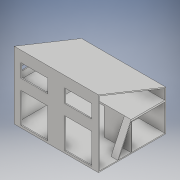
# Autodesk Inventor part: out
Saved by Autodesk Inventor 2017 (Build 210142000, 142)
## iProperties
Created: 2019-10-04
Part Number: out
Material: Generic
Document SubType Name: Modeling
Designer: Ellie
Density: 1 g/cm^3
Appearance: Default
Author: Ellie
Autodesk Inventor part; units mm, degrees
ref_plane "YZ Plane" through (0, 0, 0) normal (1, 0, 0) x (0, 1, 0)
ref_plane "XZ Plane" through (0, 0, 0) normal (0, 1, 0) x (-1, 0, 0)
sketch "Sketch1" plane through (0, 0, 0) normal (0, 1, 0) x (-1, 0, 0)
  line L0 (-3048, 3810) -> (3048, 3810)
  line L1 (3048, 3810) -> (3048, -3810)
  line L2 (3048, -3810) -> (-3048, -3810)
  line L3 (-3048, -3810) -> (-3048, 3810)
  line L4 (-3048, 3810) -> (3048, -3810) construction
  line L5 (3048, 3810) -> (-3048, -3810) construction
  point P0 (0, 0)
  dimension "d0" = 7620
  dimension "d1" = 6096
  constraints: 12 end point, 2 midpoint, 2 parallel, 1 horizontal, 1 perpendicular
  measures "d0" distance of L0.end L1.end
  measures "d1" distance of L1.end L2.end
extrude "main body" add sketch "Sketch1" along normal blind 3657.6
sketch "Sketch3" plane through (0, 0, 0) normal (0, 0, 1) x (1, 0, 0)
  line L0 (-3048, 3657.6) -> (-3048, 6096)
  line L1 (-3048, 6096) -> (3048, 3657.6)
  line L2 (3048, 3657.6) -> (-3048, 3657.6)
  point P0 (0, 0)
  dimension "d4" = 2438.4
  constraints: 6 end point, 2 coincident, 1 vertical
  measures "d4" distance of L0.start L0.end
extrude "triangle" add sketch "Sketch3" along normal mid plane 7620
shell "Shell1" thickness 88.9 removed faces 1 at (-1016, 3251.2, 3810)
ref_plane "Work Plane1" through (-2959.1, 2527.3, 3810) normal (0, 1, 0) x (1, 0, 0)
sketch "Sketch6" plane through (-2959.1, 2527.3, 3810) normal (0, 1, 0) x (1, 0, 0)
  line L0 (5918.2, 0) -> (2870.2, 0)
  line L1 (2870.2, 0) -> (2870.2, 7531.1)
  line L2 (2870.2, 7531.1) -> (5918.2, 7531.1)
  line L3 (5918.2, 7531.1) -> (5918.2, 0)
  point P0 (2959.1, 3810)
  dimension "d12" = 3048
  constraints: 8 end point, 2 parallel, 1 coincident, 1 horizontal, 1 perpendicular
  measures "d12" distance of L0.start L0.end
extrude "second floor" add sketch "Sketch6" along normal blind 152.4
ref_plane "Work Plane3" through (-2959.1, 3136.9, 3810) normal (0, 1, 0) x (1, 0, 0)
sketch "Sketch8" plane through (-2959.1, 3136.9, 3810) normal (0, 1, 0) x (1, 0, 0)
  line L0 (0, 7531.1) -> (2870.2, 7531.1)
  line L1 (2870.2, 7531.1) -> (2870.2, 5397.5)
  line L2 (2870.2, 5397.5) -> (0, 5397.5)
  line L3 (0, 5397.5) -> (0, 7531.1)
  line L4 (2870.2, 7531.1) -> (2870.2, 0) projected
  line L5 (0, 0) -> (0, 7531.1) projected
  line L6 (2870.2, 7531.1) -> (3479.8, 7531.1)
  line L7 (3479.8, 7531.1) -> (3479.8, 6616.7)
  line L8 (3479.8, 6616.7) -> (2870.2, 6616.7)
  line L9 (2870.2, 6616.7) -> (2870.2, 7531.1)
  point P0 (2959.1, 3810)
  dimension "d17" = 0
  dimension "d19" = 0
  dimension "d20" = 2133.6
  dimension "d23" = 0
  dimension "d39" = 609.6
  dimension "d40" = 914.4
  constraints: 16 end point, 4 parallel, 2 horizontal, 2 perpendicular, 1 collinear
  measures "d17" distance between parallel lines of L4 L1
  measures "d19" distance from line of L0 L5.end
  measures "d20" distance of L0.end L1.end
  measures "d23" distance between parallel lines of L5 L3
  measures "d39" distance of L7.end L8.end
  measures "d40" distance of L6.end L7.end
extrude "bedroom" add sketch "Sketch8" along normal blind 152.4
sketch "Sketch16" plane through (-88.9, 3136.9, -1587.5) normal (1, 0, 0) x (0, 0, -1)
  line L0 (1219.2, 0) -> (304.8, -457.2)
  line L1 (1219.2, 0) -> (1219.2, 152.4) projected
  line L2 (2133.6, -457.2) -> (-5397.5, -457.2) projected
  line L3 (0, 0) -> (0, 152.4) projected
  line L4 (1219.2, 152.4) -> (0, -457.2)
  line L5 (2133.6, -457.2) -> (-5397.5, -457.2) projected
  line L6 (304.8, -457.2) -> (0, -457.2)
  line L7 (1219.2, 152.4) -> (1219.2, 0)
  point P0 (-1587.5, -3136.9)
  point P1 (-1803.4, -558.8)
  point P2 (-5397.5, -457.2)
  dimension "d42" = 0
  constraints: 8 end point, 1 horizontal, 1 parallel, 1 vertical, 4 other
  measures "d42" distance from line of L3 L4.end
extrude "upper stairs" add sketch "Sketch16" along normal blind 609.6
sketch "Sketch17" plane through (-3048, 0, 3810) normal (0, 0, 1) x (1, 0, 0)
  line L0 (2959.1, 2527.3) -> (1822.0554, 88.9)
  line L1 (6007.1, 88.9) -> (88.9, 88.9) projected
  line L2 (2959.1, 2679.7) -> (1750.9901, 88.9)
  line L3 (6007.1, 2527.3) -> (2959.1, 2527.3) projected
  line L4 (3022.6, 2527.3) -> (3022.6, 25.4) projected
  line L5 (2959.1, 2679.7) -> (2959.1, 2527.3)
  line L6 (1750.9901, 88.9) -> (1822.0554, 88.9)
  line L7 (2959.1, 2679.7) -> (6007.1, 2679.7) projected
  line L8 (2959.1, 2527.3) -> (2959.1, 2679.7) projected
  line L9 (2959.1, 2679.7) -> (2959.1, 2527.3)
  point P0 (3048, 0)
  point P1 (88.9, 88.9)
  point P2 (3022.6, 25.4)
  dimension "d46" = 115
  constraints: 10 end point, 1 coincident, 1 collinear, 1 horizontal, 1 parallel, 1 vertical, 3 other
  measures "d46" angle of L3 L0
extrude "main stairs" add sketch "Sketch17" against normal blind 609.6 contours L0 L1 L2 L5
sketch "Sketch18" plane through (2959.1, 88.9, -3721.1) normal (-1, 0, 0) x (0, 0, 1)
  point P0 (3721.1, -88.9)
ref_plane "Work Plane4" through (0, 0, 1371.6) normal (0, 0, 1) x (1, 0, 0)
sketch "Sketch20" plane through (0, 0, 1371.6) normal (0, 0, 1) x (1, 0, 0)
  line L0 (2959.1, 2527.3) -> (-88.9, 2527.3) projected
  line L1 (2959.1, 88.9) -> (2959.1, 2527.3) projected
  line L2 (-88.9, 2527.3) -> (2959.1, 2527.3)
  line L3 (2959.1, 2527.3) -> (2959.1, 88.9)
  line L4 (2959.1, 88.9) -> (-88.9, 88.9)
  line L5 (-88.9, 88.9) -> (-88.9, 2527.3)
  point P0 (0, 0)
  constraints: 8 end point, 2 parallel, 1 horizontal, 1 perpendicular
extrude "room wall 1" add sketch "Sketch20" along normal blind 50.8
sketch "Sketch21" plane through (-88.9, 2679.7, -3721.1) normal (-1, 0, 0) x (0, 0, 1)
  line L0 (7531.1, -152.4) -> (5143.5, -152.4) projected
  line L1 (5143.5, -2590.8) -> (7531.1, -2590.8) projected
  line L2 (5143.5, -152.4) -> (7531.1, -152.4)
  line L3 (7531.1, -152.4) -> (7531.1, -2590.8)
  line L4 (7531.1, -2590.8) -> (5143.5, -2590.8)
  line L5 (5143.5, -2590.8) -> (5143.5, -152.4)
  line L6 (6921.5, -2590.8) -> (6921.5, 0) projected
  line L7 (5143.5, -152.4) -> (5143.5, -2590.8) projected
  point P0 (3721.1, -2679.7)
  constraints: 8 end point, 3 parallel, 2 point on line, 1 horizontal
extrude "room wall 2" add sketch "Sketch21" against normal blind 50.8
sketch "Sketch23" plane through (-3048, 0, 3810) normal (0, 0, 1) x (1, 0, 0)
  line L0 (0, 0) -> (0, 6096) projected
  line L1 (6096, 0) -> (6096, 3657.6) projected
  line L2 (0, 6096) -> (6096, 3657.6)
  line L3 (6096, 3657.6) -> (6096, 0)
  line L4 (6096, 0) -> (0, 0) projected
  line L5 (6096, 0) -> (0, 0)
  line L6 (6096, 3657.6) -> (0, 6096) projected
  line L7 (0, 0) -> (0, 6096)
  line L8 (1750.9901, 88.9) -> (88.9, 88.9) projected
  point P0 (3048, 0)
  point P1 (88.9, 5964.6918)
  point P2 (6007.1, 3597.4118)
  point P3 (6007.1, 88.9)
  constraints: 8 end point, 2 perpendicular, 1 collinear
extrude "outer wall" [suppressed]
sketch "Sketch24" plane through (-3048, 0, -3810) normal (-1, 0, 0) x (0, 0, 1)
  line L0 (609.6, 2946.4) -> (3048, 2946.4)
  line L1 (3048, 2946.4) -> (3048, 203.2)
  line L2 (3048, 203.2) -> (609.6, 203.2)
  line L3 (609.6, 203.2) -> (609.6, 2946.4)
  line L4 (7620, 0) -> (0, 0) projected
  line L5 (0, 0) -> (0, 6096) projected
  line L6 (7620, 0) -> (7620, 6096) projected
  line L7 (4572, 2946.4) -> (7010.4, 2946.4)
  line L8 (7010.4, 2946.4) -> (7010.4, 203.2)
  line L9 (7010.4, 203.2) -> (4572, 203.2)
  line L10 (4572, 203.2) -> (4572, 2946.4)
  line L11 (2222.5, 3289.3) -> (88.9, 3289.3) projected
  point P0 (3810, 0)
  point P1 (3810, 0)
  dimension "d62" = 203.2
  dimension "d63" = 2438.4
  dimension "d64" = 609.6
  dimension "d65" = 2743.2
  dimension "d73" = 203.2
  dimension "d74" = 609.6
  constraints: 16 end point, 4 parallel, 2 equal length, 2 horizontal, 2 perpendicular, 1 midpoint
  measures "d62" distance between parallel lines of L4 L2
  measures "d63" distance of L0.start L0.end
  measures "d64" distance between parallel lines of L5 L3
  measures "d65" distance of L0.end L1.end
  measures "d73" distance between parallel lines of L4 L9
  measures "d74" distance between parallel lines of L6 L8
sketch "Sketch26" plane through (3048, 0, -3810) normal (0, 0, -1) x (-1, 0, 0)
  line L0 (4787.9, 4308.729) -> (5702.3, 4308.729)
  line L1 (5702.3, 4308.729) -> (5702.3, 3898.9)
  line L2 (5702.3, 3898.9) -> (4787.9, 3898.9)
  line L3 (4787.9, 3898.9) -> (4787.9, 4308.729)
  line L4 (3136.9, 3136.9) -> (6007.1, 3136.9) projected
  line L5 (6007.1, 3289.3) -> (6007.1, 5964.6918) projected
  line L6 (6007.1, 3289.3) -> (2527.3, 3289.3) projected
  point P0 (3048, 0)
  dimension "d78" = 914.4
  dimension "d79" = 409.829
  dimension "d81" = 304.8
  dimension "d95" = 609.6
  constraints: 8 end point, 2 parallel, 1 horizontal, 1 perpendicular
  measures "d78" distance of L0.start L0.end
  measures "d79" distance of L0.end L1.end
  measures "d81" distance between parallel lines of L5 L1
  measures "d95" distance between parallel lines of L6 L2
extrude "side window 1" cut sketch "Sketch26" against normal up to next
sketch "Sketch30" plane through (-3048, 0, -3810) normal (-1, 0, 0) x (0, 0, 1)
  line L0 (609.6, 5118.1) -> (3048, 5118.1)
  line L1 (3048, 5118.1) -> (3048, 3898.9)
  line L2 (3048, 3898.9) -> (609.6, 3898.9)
  line L3 (609.6, 3898.9) -> (609.6, 5118.1)
  line L4 (0, 4308.729) -> (0, 3898.9) projected
  line L5 (2222.5, 3289.3) -> (88.9, 3289.3) projected
  line L6 (0, 0) -> (0, 6096) projected
  line L7 (7620, 0) -> (7620, 6096) projected
  line L8 (4572, 3898.9) -> (4572, 5118.1)
  line L9 (4572, 5118.1) -> (7010.4, 5118.1)
  line L10 (7010.4, 5118.1) -> (7010.4, 3898.9)
  line L11 (7010.4, 3898.9) -> (4572, 3898.9)
  point P0 (3810, 0)
  dimension "d105" = 2438.4
  dimension "d106" = 609.6
  dimension "d107" = 609.6
  dimension "d118" = 1219.2
  dimension "d121" = 3962.4
  constraints: 16 end point, 2 horizontal, 2 parallel, 1 perpendicular, 8 other
  measures "d105" distance of L0.start L0.end
  measures "d106" distance between parallel lines of L5 L2
  measures "d107" distance between parallel lines of L6 L3
  measures "d118" distance of L0.end L1.end
  measures "d121" distance of L2.end L8.start
sketch "Sketch28" plane through (-3048, 0, 3810) normal (0, 0, 1) x (1, 0, 0)
  line L0 (0, 0) -> (0, 6096) projected
  line L1 (0, 6096) -> (6096, 3657.6) projected
  line L2 (0, 6096) -> (6096, 3657.6)
  line L3 (6096, 0) -> (0, 0) projected
  line L4 (6096, 3657.6) -> (6096, 0)
  line L5 (6096, 0) -> (0, 0)
  line L6 (0, 0) -> (0, 6096)
  point P0 (3048, 0)
  constraints: 8 end point, 3 perpendicular, 1 collinear
extrude "my WALL" [suppressed]
sketch "Sketch29" plane through (-3048, 0, 3810) normal (0, 0, 1) x (1, 0, 0)
  line L0 (393.7, 3898.9) -> (393.7, 4308.729) projected
  line L1 (393.7, 3898.9) -> (1308.1, 3898.9) projected
  line L2 (393.7, 4308.729) -> (1308.1, 4308.729)
  line L3 (1308.1, 4308.729) -> (1308.1, 3898.9)
  line L4 (1308.1, 3898.9) -> (393.7, 3898.9)
  line L5 (393.7, 3898.9) -> (393.7, 4308.729)
  point P0 (3048, 0)
  constraints: 8 end point, 2 parallel, 1 horizontal, 1 perpendicular
extrude "other side window 1" [suppressed]
extrude "front bottom windows" cut sketch "Sketch24" against normal up to next
extrude "front top windows" cut sketch "Sketch30" against normal up to next
equation "\"d73\" = d62"
body "Solid1"
